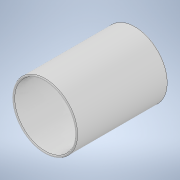
# Autodesk Inventor part: Part1
Saved by Autodesk Inventor 2022.2 (Build 262287000, 287)
## iProperties
Created: 2022-09-08
Part Number: Part1
Material: Generic
Document SubType Name: Modeling
Designer: Andrei
Density: 1 g/cm^3
Appearance: Default
Author: Andrei
Autodesk Inventor part; units mm, degrees
ref_plane "YZ Plane" through (0, 0, 0) normal (1, 0, 0) x (0, 1, 0)
ref_plane "XZ Plane" through (0, 0, 0) normal (0, 1, 0) x (-1, 0, 0)
ref_plane "XY Plane" through (0, 0, 0) normal (0, 0, 1) x (1, 0, 0)
sketch "Sketch1" plane through (0, 0, 0) normal (0, 0, 1) x (1, 0, 0)
  circle A0 centre (0, 0) radius 42.5
  circle A1 centre (0, 0) radius 40
  dimension "d0" = 85
  dimension "d1" = 80
  constraints: 2 centre point, 2 coincident
  measures "d0" diameter of A0
  measures "d1" diameter of A1
extrude "Extrusion1" add sketch "Sketch1" along normal blind 120
fillet "Fillet1" radius 1.25 1 edges at (-42.5, 0, 120)
fillet "Fillet2" radius 1.25 1 edges at (-42.5, 0, 0)
fillet "Fillet3" radius 1.25 1 edges at (-40, 0, 0)
fillet "Fillet4" radius 1.25 1 edges at (-40, 0, 120)
equation "\"d0\" = OuterDiameter"
equation "\"d1\" = InnerDiameter"
equation "\"d2\" = height"
equation "\"d4\" = fillet"
equation "\"d5\" = fillet"
equation "\"d6\" = fillet"
equation "\"d7\" = fillet"
equation "\"OuterDiameter\" = InnerDiameter + thickness"
equation "\"InnerDiameter\" = 80"
equation "\"thickness\" = 5"
equation "\"height\" = 120"
equation "\"fillet\" = 0.25 * thickness"
body "Solid1"
